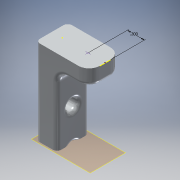
# Autodesk Inventor part: LidSupportLW
Saved by Autodesk Inventor 2016 (Build 200138000, 138)
## iProperties
Created: 2015-07-14
Part Number: LidSupportLW
Material: Generic
Document SubType Name: Modeling
Designer: Karl
Density: 1 g/cm^3
Appearance: Default
Author: Karl
Autodesk Inventor part; units mm, degrees
ref_plane "YZ Plane" through (0, 0, 0) normal (1, 0, 0) x (0, 1, 0)
ref_plane "XZ Plane" through (0, 0, 0) normal (0, 1, 0) x (-1, 0, 0)
ref_plane "XY Plane" through (0, 0, 0) normal (0, 0, 1) x (1, 0, 0)
sketch "Sketch1" plane through (0, 0, 0) normal (0, 1, 0) x (-1, 0, 0)
  line L0 (3.175, -4.7625) -> (-3.175, -4.7625)
  line L1 (-3.175, -4.7625) -> (-3.175, 4.7625)
  line L2 (-3.175, 4.7625) -> (3.175, 4.7625)
  line L3 (3.175, 4.7625) -> (3.175, -4.7625)
  line L4 (3.175, -4.7625) -> (-3.175, 4.7625) construction
  line L5 (-3.175, -4.7625) -> (3.175, 4.7625) construction
  point P0 (0, 0)
  point P1 (0, 0)
  point P2 (0, 0)
  point P3 (0, 0)
  dimension "d0" = 9.525
  dimension "d1" = 6.35
  constraints: 12 end point, 4 midpoint, 2 coincident, 2 parallel, 1 horizontal, 1 perpendicular
  measures "d0" distance of L0.end L1.end
  measures "d1" distance of L1.end L2.end
extrude "Extrusion1" add sketch "Sketch1" along normal blind 120.65
sketch "Sketch2" plane through (0, 0, 0) normal (0, -1, 0) x (1, 0, 0)
  line L0 (3.175, 4.7625) -> (12.7, 4.7625)
  line L1 (12.7, 4.7625) -> (12.7, -4.7625)
  line L2 (12.7, -4.7625) -> (3.175, -4.7625)
  line L3 (3.175, -4.7625) -> (3.175, 4.7625)
  point P0 (0, 0)
  dimension "d4" = 9.525
  constraints: 8 end point, 2 parallel, 1 horizontal, 1 perpendicular
  measures "d4" distance of L1.end L2.end
extrude "Extrusion2" add sketch "Sketch2" against normal blind 4.7625
sketch "Sketch3" plane through (0, 120.65, 0) normal (0, 1, 0) x (1, 0, 0)
  line L0 (3.175, -4.7625) -> (3.175, 4.7625) projected
  line L1 (3.175, -4.7625) -> (12.7, -4.7625) projected
  line L2 (12.7, -4.7625) -> (12.7, 4.7625) projected
  line L3 (12.7, 4.7625) -> (3.175, 4.7625) projected
  point P0 (0, 0)
extrude "Extrusion3" add sketch "Sketch3" against normal blind 4.7625
fillet "Fillet1" radius 3.175 4 edges at (12.7, 2.3813, -4.7625) (12.7, 2.3813, 4.7625) (12.7, 118.2687, -4.7625) (12.7, 118.2687, 4.7625)
fillet "Fillet2" radius 3.175 2 edges at (3.175, 4.7625, 0) (3.175, 115.8875, 0)
fillet "Fillet3" radius 1.27 12 edges at (7.9375, 115.8875, -4.7625) (11.7701, 115.8875, -3.8326) (12.7, 115.8875, 0) (11.7701, 115.8875, 3.8326) (7.9375, 115.8875, 4.7625) (3.175, 60.325, 4.7625) (7.9375, 4.7625, 4.7625) (11.7701, 4.7625, 3.8326) (12.7, 4.7625, 0) (11.7701, 4.7625, -3.8326) (7.9375, 4.7625, -4.7625) (3.175, 60.325, -4.7625)
sketch "Sketch7" plane through (3.175, 7.9375, 3.4925) normal (1, 0, 0) x (0, 0, -1)
  line L0 (0, 0) -> (0, 104.775) projected
  line L1 (5.08, -7.9375) -> (1.905, -7.9375) projected
  line L2 (0, 52.3875) -> (19.363, 52.3875)
  point P0 (3.4925, -7.9375)
  point P1 (3.4925, 7.9375)
  point P2 (3.4925, 30.1625)
  point P3 (3.4925, 52.3875)
  point P4 (3.4925, 96.8375)
  point P5 (3.4925, 74.6125)
  point P6 (3.4925, 19.05)
  point P7 (3.4925, 41.275)
  point P8 (3.4925, 85.725)
  point P9 (3.4925, 63.5)
  dimension "d25" = 15.875
  dimension "d26" = 22.225
  dimension "d27" = 11.1125
  dimension "d28" = 11.1125
  constraints: 4 symmetric about line, 2 end point, 1 midpoint, 1 parallel, 1 point on line
  measures "d25" distance from line of L1 point (3.492, 7.938)
  measures "d26" distance of point (3.493, 30.163) point (3.492, 7.938)
  measures "d27" distance of point (3.492, 19.05) point (3.492, 7.938)
  measures "d28" distance of point (3.492, 41.275) point (3.493, 30.163)
hole "Hole2" at (3.175, 15.875, 0) at (3.175, 38.1, 0) at (3.175, 60.325, 0) at (3.175, 82.55, 0) at (3.175, 104.775, 0) at (3.175, 26.9875, 0) at (3.175, 49.2125, 0) at (3.175, 93.6625, 0) at (3.175, 71.4375, 0) direction (-1, 0, 0) diameter 3.175 depth 203.2 tip angle 118
fillet "Fillet4" radius 1.27 9 edges at (3.175, 104.775, 1.5875) (3.175, 93.6625, 1.5875) (3.175, 82.55, 1.5875) (3.175, 71.4375, 1.5875) (3.175, 60.325, 1.5875) (3.175, 49.2125, 1.5875) (3.175, 38.1, 1.5875) (3.175, 26.9875, 1.5875) (3.175, 15.875, 1.5875)
fillet "Fillet5" radius 1.27 9 edges at (-3.175, 104.775, 1.5875) (-3.175, 93.6625, 1.5875) (-3.175, 82.55, 1.5875) (-3.175, 71.4375, 1.5875) (-3.175, 60.325, 1.5875) (-3.175, 49.2125, 1.5875) (-3.175, 38.1, 1.5875) (-3.175, 26.9875, 1.5875) (-3.175, 15.875, 1.5875)
fillet "Fillet6" radius 1.27 2 edges at (-3.175, 60.325, -4.7625) (-3.175, 60.325, 4.7625)
sketch "Sketch4" plane through (0, 120.65, 0) normal (0, 1, 0) x (1, 0, 0)
  line L0 (12.7, -1.5875) -> (12.7, 1.5875) projected
  point P0 (0, 0)
  point P1 (7.62, 0)
  point P2 (12.7, 0)
  dimension "d11" = 5.08
  constraints: 1 horizontal alignment, 1 midpoint
  measures "d11" distance from line of L0 point (7.62, 0)
ref_plane "Work Plane3" through (0, 95.25, 0) normal (0, 1, 0) x (1, 0, 0)
sketch "Sketch11" plane through (0, 95.25, 0) normal (0, 1, 0) x (1, 0, 0)
  line L0 (-3.175, 4.7625) -> (12.7, 4.7625)
  line L1 (12.7, 4.7625) -> (12.7, -4.7625)
  line L2 (12.7, -4.7625) -> (-3.175, -4.7625)
  line L3 (-3.175, -4.7625) -> (-3.175, 4.7625)
  arc A0 (-3.175, -3.4925) -> (-1.905, -4.7625) centre (-1.905, -3.4925) ccw projected
  line L4 (-3.175, -3.4925) -> (-3.175, 3.4925) projected
  arc A1 (-1.905, 4.7625) -> (-3.175, 3.4925) centre (-1.905, 3.4925) ccw projected
  line L5 (-1.905, 4.7625) -> (9.525, 4.7625) projected
  arc A2 (12.7, 1.5875) -> (9.525, 4.7625) centre (9.525, 1.5875) ccw projected
  line L6 (12.7, 1.5875) -> (12.7, -1.5875) projected
  arc A3 (9.525, -4.7625) -> (12.7, -1.5875) centre (9.525, -1.5875) ccw projected
  line L7 (9.525, -4.7625) -> (-1.905, -4.7625) projected
  point P0 (0, 0)
  constraints: 8 end point, 4 collinear, 2 parallel, 1 horizontal, 1 perpendicular
extrude "Extrusion10" cut sketch "Sketch11" against normal through all contours L0 A2 L1 A3 L2 A0 L3 A1
body "Solid1"
